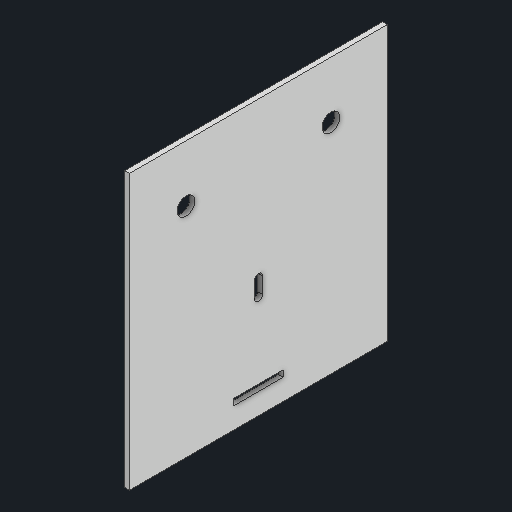
# Autodesk Inventor part: test_rig_plate
Saved by Autodesk Inventor 2027.1 (Build 311270010, 270A)
## iProperties
Created: 2026-09-04
Part Number: test_rig_plate
Material: Generic
Document SubType Name: Modeling
Designer: ajrcr
Density: 1 g/cm^3
Appearance: Default
Author: ajrcr
Autodesk Inventor part; units mm, degrees
ref_plane "YZ Plane" through (0, 0, 0) normal (1, 0, 0) x (0, 1, 0)
ref_plane "XZ Plane" through (0, 0, 0) normal (0, 1, 0) x (-1, 0, 0)
ref_plane "XY Plane" through (0, 0, 0) normal (0, 0, 1) x (1, 0, 0)
sketch "Sketch1" plane through (0, 0, 0) normal (1, 0, 0) x (0, 1, 0)
  ellipse E0 centre (-0.5259, 43.2954) end of major axis (4.9729, 43.4114) minor radius 5.4993 projected
  ellipse E1 centre (-0.5259, 43.2954) end of major axis (34.4663, 44.0334) minor radius 34.9957 construction
  ellipse E2 centre (-0.4397, -46.3999) end of major axis (4.5348, -48.7461) minor radius 5.5 projected
  ellipse E3 centre (-0.4397, -46.3999) end of major axis (31.2162, -61.3299) minor radius 35 construction
  line L0 (34.4741, 78.2911) -> (34.4741, -81.3999)
  line L1 (34.4741, -81.3999) -> (-135.3535, -81.3999)
  line L2 (-135.3535, -81.3999) -> (-135.3535, -41.4232)
  line L3 (-135.3535, -41.4232) -> (-135.3535, 29.6374)
  line L4 (-135.3535, 29.6374) -> (-135.3535, 78.2911)
  line L5 (-135.3535, 78.2911) -> (34.4741, 78.2911)
  line L6 (34.4741, 78.2911) -> (-35.4397, 78.2911) construction
  line L7 (-35.4397, 78.2911) -> (-35.4397, -81.3999) construction
  line L8 (-35.4397, -81.3999) -> (34.4741, -81.3999) construction
  line L9 (34.4741, -81.3999) -> (34.4741, 78.2911) construction
  line L10 (-0.5259, 43.2954) -> (-0.4397, -46.3999) construction
  line L11 (-0.4828, -1.5523) -> (-135.3535, -1.5523) construction
  line L12 (-61.5269, -1.5523) -> (-71.5269, -1.5523) construction
  line L13 (-61.5269, 0.9477) -> (-71.5269, 0.9477)
  line L14 (-71.5269, -4.0523) -> (-61.5269, -4.0523)
  arc A0 (-61.5269, -4.0523) -> (-61.5269, 0.9477) centre (-61.5269, -1.5523) ccw
  arc A1 (-71.5269, 0.9477) -> (-71.5269, -4.0523) centre (-71.5269, -1.5523) ccw
  ellipse E4 centre (-0.5269, 43.3424) end of major axis (-30.5202, 42.7098) minor radius 29.9963 construction
  line L15 (-30.5269, 78.2911) -> (-30.5269, -81.3999) construction
  line L16 (-118.3535, 13.7477) -> (-122.3535, 13.7477)
  line L17 (-122.3535, 13.7477) -> (-122.3535, -16.8523)
  line L18 (-122.3535, -16.8523) -> (-118.3535, -16.8523)
  line L19 (-118.3535, -16.8523) -> (-118.3535, 13.7477)
  line L20 (-118.3535, 13.7477) -> (-122.3535, -16.8523) construction
  line L21 (-122.3535, 13.7477) -> (-118.3535, -16.8523) construction
  point P0 (0, 0)
  point P1 (-66.5269, -1.5523)
  point P2 (-120.3535, -1.5523)
  dimension "d1" = 69.9138
  dimension "d2" = 169.8276
  dimension "d3" = 5
  dimension "d4" = 36
  dimension "d5" = 10
  dimension "d8" = 4
  dimension "d9" = 30.6
  dimension "d10" = 15
  constraints: 46 end point, 8 parallel, 6 point on line, 5 perpendicular, 4 collinear, 4 midpoint, 4 point on circle, 4 tangent, 3 horizontal, 2 centre point, 2 vertical, 5 other
  measures "d1" distance between parallel lines of L0 L7
  measures "d2" distance of L4.end L0.start
  measures "d3" diameter of A1
  measures "d4" distance from line of point (-66.527, -1.552) L15
  measures "d5" distance of L12.start L12.end
  measures "d8" distance of L18.end L17.end
  measures "d9" distance of L17.end L16.end
  measures "d10" distance from line of point (-120.354, -1.552) L3
extrude "Extrusion1" add sketch "Sketch1" along normal blind 3
body "Solid1"
